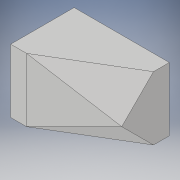
# Autodesk Inventor part: 零件16
Saved by Autodesk Inventor 2019 (Build 230136000, 136)
## iProperties
Created: 2020-09-18
Part Number: 零件16
Material: 一般
Document SubType Name: Modeling
Designer: jay
Density: 1 g/cm^3
Appearance: 預設
Author: jay
Autodesk Inventor part; units mm, degrees
ref_plane "YZ Plane" through (0, 0, 0) normal (1, 0, 0) x (0, 1, 0)
sketch "草圖1" plane through (0, 0, 0) normal (0, 0, 1) x (1, 0, 0)
  line L0 (0, 0) -> (60, 0)
  line L1 (60, 0) -> (60, 40)
  line L2 (60, 40) -> (0, 40)
  line L3 (0, 40) -> (0, 0)
  dimension "d0" = 60
  dimension "d1" = 40
  constraints: 8 end point, 2 parallel, 1 horizontal, 1 perpendicular
  measures "d0" distance of L1.end L2.end
  measures "d1" distance of L0.end L1.end
extrude "擠出1" add sketch "草圖1" along normal blind 40
chamfer "倒角1" distance 50 distance2 10 1 edges at (60, 20, 40) measured on face at (20, 26.6667, 40)
sketch "草圖2" plane through (60, 0, 0) normal (1, 0, 0) x (0, 0, -1)
  line L0 (0, 40) -> (-30, 40) projected
  line L1 (0, 0) -> (0, 40) projected
  line L2 (0, 0) -> (-30, 0) projected
  line L3 (-40, 40) -> (-40, 0) projected
  point P0 (-10, 40)
  point P1 (-10, 0)
  point P2 (-40, 20)
  dimension "d7" = 10
  dimension "d10" = 10
  dimension "d13" = 20
  constraints: 2 point on line, 1 midpoint
  measures "d7" distance from line of L1 point (-10, 40)
  measures "d10" distance from line of L1 point (-10, 0)
  measures "d13" distance from line of L2 point (-40, 20)
ref_plane "工作平面3" through (60, 40, 10) normal (-0.3906, -0.6509, -0.6509) x (0, -0.7071, 0.7071)
ref_plane "工作平面4" through (60, 20, 30) normal (-0.3906, 0.6509, -0.6509) x (0, -0.7071, -0.7071)
sketch "草圖5" plane through (60, 40, 10) normal (-0.3906, -0.6509, -0.6509) x (0, -0.7071, 0.7071)
  line L0 (-21.2028, 86.012) -> (46.7944, 86.012)
  line L1 (46.7944, 86.012) -> (46.7944, -28.5442)
  line L2 (46.7944, -28.5442) -> (-21.2028, -28.5442)
  line L3 (-21.2028, -28.5442) -> (-21.2028, 86.012)
  point P0 (21.2132, 41.4259)
  constraints: 8 end point, 2 parallel, 1 horizontal, 1 perpendicular
extrude "擠出4" cut sketch "草圖5" against normal blind 40
sketch "草圖6" plane through (60, 20, 30) normal (-0.3906, 0.6509, -0.6509) x (0, -0.7071, -0.7071)
  line L0 (-21.2652, 80.224) -> (44.7592, 80.224)
  line L1 (44.7592, 80.224) -> (44.7592, -31.1757)
  line L2 (44.7592, -31.1757) -> (-21.2652, -31.1757)
  line L3 (-21.2652, -31.1757) -> (-21.2652, 80.224)
  point P0 (35.3553, 52.4728)
  constraints: 8 end point, 2 parallel, 1 horizontal, 1 perpendicular
extrude "擠出5" cut sketch "草圖6" against normal blind 40
